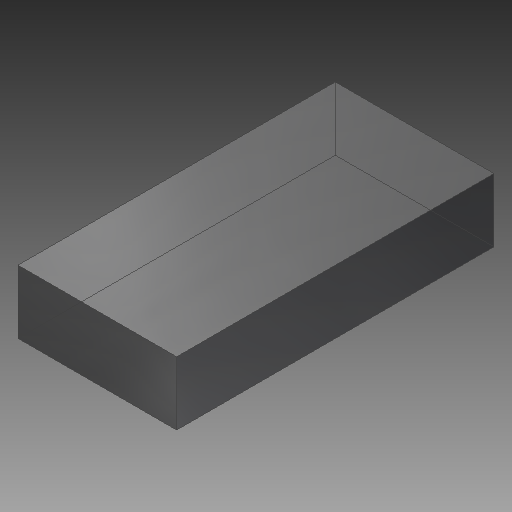
# Autodesk Inventor part: Gelpad 10x5
Saved by Autodesk Inventor 2019.1 (Build 231200000, 200)
## iProperties
Created: 2015-08-25
Part Number: Gelpad 10x5
Material: Gummi, Silikon
Document SubType Name: Modeling
Designer: ryll
Mass: 0.125 g
Surface Area: 1.6 cm^2
Volume: 0.1 cm^3
Density: 1.25 g/cm^3
Appearance: Gummi - schwarz - Version 1.1
Author: ryll
Autodesk Inventor part; units mm, degrees
ref_plane "YZ Plane" through (0, 0, 0) normal (1, 0, 0) x (0, 1, 0)
ref_plane "XZ Plane" through (0, 0, 0) normal (0, 1, 0) x (-1, 0, 0)
ref_plane "XY Plane" through (0, 0, 0) normal (0, 0, 1) x (1, 0, 0)
sketch "Skizze1" plane through (0, 0, 0) normal (0, 0, 1) x (1, 0, 0)
  line L0 (-2.5, 5) -> (2.5, 5)
  line L1 (2.5, 5) -> (2.5, -5)
  line L2 (2.5, -5) -> (-2.5, -5)
  line L3 (-2.5, -5) -> (-2.5, 5)
  line L4 (-3.5, 0) -> (3.5, 0) projected
  line L5 (0, 7) -> (0, -7) projected
  point P0 (0, 0)
  dimension "d0" = 5
  dimension "d1" = 10
  constraints: 8 end point, 2 parallel, 1 horizontal, 1 perpendicular, 2 other
  measures "d0" distance of L0.start L0.end
  measures "d1" distance of L0.end L1.end
extrude "Extrusion1" add sketch "Skizze1" along normal blind 2
